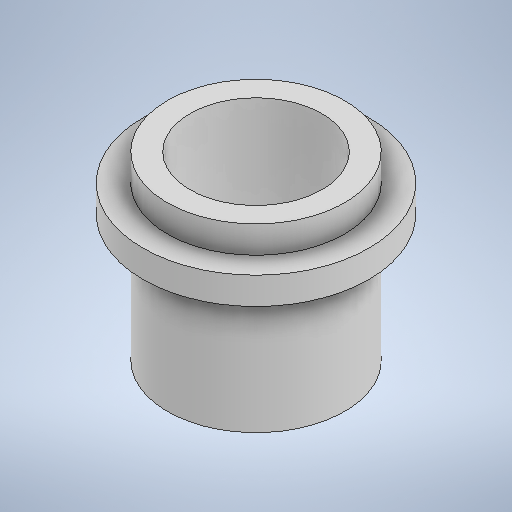
# Autodesk Inventor part: Pomodoro Robot Neck
Saved by Autodesk Inventor 2025.3 (Build 293356030, 356C)
## iProperties
Created: 2026-07-20
Part Number: Pomodoro Robot Neck
Material: Generic
Document SubType Name: Modeling
Designer: Samuel Correa Vega
Density: 1 g/cm^3
Appearance: Default
Author: Samuel Correa Vega
Autodesk Inventor part; units mm, degrees
ref_plane "YZ Plane" through (0, 0, 0) normal (1, 0, 0) x (0, 1, 0)
ref_plane "XZ Plane" through (0, 0, 0) normal (0, 1, 0) x (-1, 0, 0)
sketch "Sketch1" plane through (0, 0, 0) normal (0, 1, 0) x (-1, 0, 0)
  circle A0 centre (0, 0) radius 9.8
  dimension "d0" = 19.6
  constraints: 1 centre point, 1 coincident
  measures "d0" diameter of A0
extrude "Extrusion1" add sketch "Sketch1" along normal blind 20
ref_plane "Work Plane1" through (0, 14, 0) normal (0, -1, 0) x (1, 0, 0)
sketch "Sketch3" plane through (0, 14, 0) normal (0, -1, 0) x (1, 0, 0)
  circle A0 centre (0, 0) radius 12.5
  dimension "d7" = 25
  constraints: 1 centre point, 1 coincident
  measures "d7" diameter of A0
extrude "Extrusion3" add sketch "Sketch3" against normal blind 3
shell "Shell1" thickness 2.5 removed faces 2 at (0.3035, 20, 2.5) at (0.3035, 0, 2.5)
body "Solid1"
